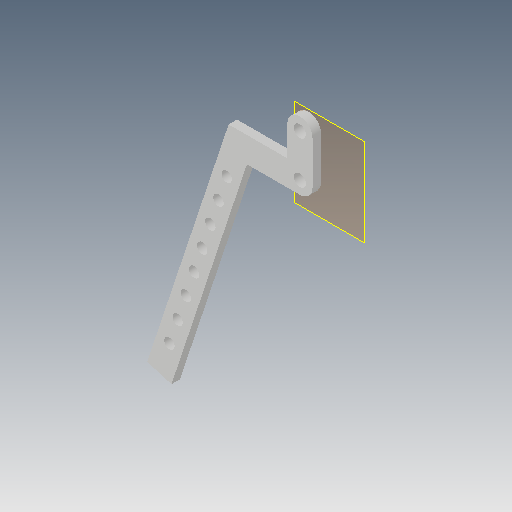
# Autodesk Inventor part: CollectorArmZ
Saved by Autodesk Inventor 2018 (Build 220112000, 112)
## iProperties
Created: 2018-12-17
Part Number: CollectorArmZ
Material: Generic
Document SubType Name: Modeling
Designer: ball
Density: 1 g/cm^3
Appearance: Default
Author: ball
Autodesk Inventor part; units mm, degrees
ref_plane "YZ Plane" through (0, 0, 0) normal (1, 0, 0) x (0, 1, 0)
ref_plane "XZ Plane" through (0, 0, 0) normal (0, 1, 0) x (-1, 0, 0)
ref_plane "XY Plane" through (0, 0, 0) normal (0, 0, 1) x (1, 0, 0)
ref_plane "Work Plane3" through (0, 0, 0) normal (0, 0, 1) x (1, 0, 0)
sketch "Sketch2" plane through (0, 0, 0) normal (0, 0, 1) x (1, 0, 0)
  arc A0 (-7.5753, -9.9544) -> (-9.0817, -9.6822) centre (-8, -8) ccw construction
  arc A1 (-9.9544, 7.5753) -> (-9.6822, 9.0817) centre (-8, 8) ccw construction
  line L0 (-8, 8) -> (-8, -8) construction
  line L1 (-3.2375, 8) -> (-3.2375, -8)
  line L2 (-12.7625, 8) -> (-12.7625, -3.2375)
  arc A2 (-3.2375, 8) -> (-12.7625, 8) centre (-8, 8) ccw
  arc A3 (-3.2375, 8) -> (-12.7625, 8) centre (-8, 8) ccw construction
  arc A4 (-8, -12.7625) -> (-3.2375, -8) centre (-8, -8) ccw
  line L3 (-76.8525, -130.4672) -> (11.0654, 135.3719) construction
  line L4 (-12.7625, -3.2375) -> (-34.7753, -3.2375)
  line L5 (-67.8092, -133.458) -> (20.1087, 132.3811) construction
  line L6 (-8, -12.7625) -> (-27.893, -12.7625)
  arc A5 (1.9836, 0.2558) -> (1.5702, -1.2387) centre (0, 0) ccw construction
  circle A6 centre (0, 0) radius 115.8748 construction
  line L7 (-34.7753, -3.2375) -> (-65.3505, -95.6884)
  line L8 (-65.3505, -95.6884) -> (-56.2232, -98.425)
  line L9 (-27.893, -12.7625) -> (-56.2232, -98.425)
  line L10 (-27.893, -12.7625) -> (-36.9363, -9.7717) construction
  line L11 (-60.7868, -97.0567) -> (-32.4146, -11.2671) construction
  circle A7 centre (-35.4852, -20.5515) radius 1.9685
  circle A8 centre (-38.5557, -29.836) radius 1.9685
  circle A9 centre (-41.6262, -39.1204) radius 1.9685
  circle A10 centre (-44.6968, -48.4048) radius 1.9685
  circle A11 centre (-47.7673, -57.6893) radius 1.9685
  circle A12 centre (-50.8378, -66.9737) radius 1.9685
  circle A13 centre (-53.9084, -76.2581) radius 1.9685
  circle A14 centre (-56.9789, -85.5426) radius 1.9685
  circle A15 centre (-8, -8) radius 2.2479
  circle A16 centre (-8, 8) radius 2.2479
  point P0 (0, 0)
  dimension "d6" = 231.7496
  dimension "d0" = 4.7625
  dimension "d1" = 4.7625
  dimension "d2" = 4.7625
  dimension "d3" = 4.7625
  dimension "d4" = 9.525
  dimension "d5" = 9.525
  dimension "d7" = 3.937
  dimension "d8" = 9.779
  dimension "d11" = 9.779
  dimension "d16" = 4.4958
  dimension "d17" = 4.4958
  constraints: 24 end point, 16 centre point, 12 point on circle, 7 point on line, 5 coincident, 3 parallel, 2 horizontal, 2 midpoint, 2 tangent, 1 perpendicular, 1 vertical, 33 other
  measures "d0" distance between parallel lines of L0 L1
  measures "d1" distance between parallel lines of L0 L2
  measures "d2" radius of A2
  measures "d3" radius of A3
  measures "d4" diameter of A4
  measures "d5" distance between parallel lines of L3 L5
  measures "d7" diameter of A7
  measures "d8" distance from line of A7.centre L10
  measures "d11" distance of A7.centre A8.centre
  measures "d16" diameter of A15
  measures "d17" diameter of A16
extrude "Extrusion1" add sketch "Sketch2" along normal blind 3.175
body "Solid1"
